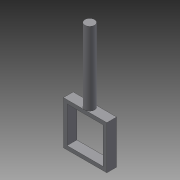
# Autodesk Inventor part: eye_cam_holder
Saved by Autodesk Inventor 2015 (Build 190159000, 159)
## iProperties
Created: 2015-06-21
Part Number: eye_cam_holder
Material: Generic
Document SubType Name: Modeling
Designer: Master
Density: 1 g/cm^3
Appearance: Default
Author: Master
Autodesk Inventor part; units mm, degrees
ref_plane "YZ Plane" through (0, 0, 0) normal (1, 0, 0) x (0, 1, 0)
ref_plane "XZ Plane" through (0, 0, 0) normal (0, 1, 0) x (-1, 0, 0)
ref_plane "XY Plane" through (0, 0, 0) normal (0, 0, 1) x (1, 0, 0)
sketch "Sketch1" plane through (0, 0, 0) normal (0, 0, 1) x (1, 0, 0)
  line L0 (8.0644, -32.7837) -> (-6.6856, -32.7837)
  line L1 (-6.6856, -32.7837) -> (-6.6856, -47.5337)
  line L2 (-6.6856, -47.5337) -> (8.0644, -47.5337)
  line L3 (8.0644, -47.5337) -> (8.0644, -32.7837)
  line L4 (9.5644, -31.2837) -> (-8.1856, -31.2837)
  line L5 (-8.1856, -31.2837) -> (-8.1856, -49.0337)
  line L6 (-8.1856, -49.0337) -> (9.5644, -49.0337)
  line L7 (9.5644, -49.0337) -> (9.5644, -31.2837)
  point P0 (0, 0)
  dimension "d0" = 1.5
  dimension "d1" = 1.5
  dimension "d2" = 1.5
  dimension "d3" = 1.5
  dimension "d4" = 14.75
  dimension "d5" = 14.75
  constraints: 16 end point
  measures "d0" distance between parallel lines of L7 L3
  measures "d1" distance between parallel lines of L6 L2
  measures "d2" distance between parallel lines of L1 L5
  measures "d3" distance between parallel lines of L0 L4
  measures "d4" distance between parallel lines of L2 L0
  measures "d5" distance between parallel lines of L1 L3
extrude "Extrusion1" add sketch "Sketch1" along normal blind 4
sketch "Sketch2" plane through (-8.1856, -31.2837, 0) normal (0, 1, 0) x (1, 0, 0)
  line L0 (17.75, 0) -> (0, 0) projected
  line L1 (0, 0) -> (0, -4) projected
  line L2 (17.75, -4) -> (0, -4) projected
  line L3 (17.75, 0) -> (17.75, -4) projected
  circle A0 centre (8.75, -2) radius 2
  point P0 (8.1856, 0)
  dimension "d8" = 4
  dimension "d9" = 9
  constraints: 1 centre point, 1 tangent
  measures "d8" diameter of A0
  measures "d9" distance from line of L3 A0.centre
extrude "Extrusion2" add sketch "Sketch2" along normal blind 30 contours A0
body "Solid1"
